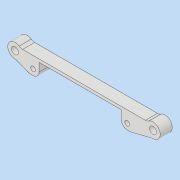
# Autodesk Inventor part: SpoolServoMount
Saved by Autodesk Inventor 2017 (Build 210142000, 142)
## iProperties
Created: 2018-04-09
Part Number: SpoolServoMount
Material: ABS Plastic
Document SubType Name: Modeling
Designer: Derek Wider
Density: 1.06 g/cm^3
Appearance: Smooth - White
Author: Derek Wider
Autodesk Inventor part; units mm, degrees
ref_plane "YZ Plane" through (0, 0, 0) normal (1, 0, 0) x (0, 1, 0)
ref_plane "XZ Plane" through (0, 0, 0) normal (0, 1, 0) x (-1, 0, 0)
ref_plane "XY Plane" through (0, 0, 0) normal (0, 0, 1) x (1, 0, 0)
sketch "Sketch1" plane through (0, 0, 0) normal (0, 0, 1) x (1, 0, 0)
  circle A0 centre (0, 0) radius 1.8415
  circle A1 centre (72.5902, 0) radius 1.8415
  line L0 (0, 0) -> (36.2951, -20.955) construction
  line L1 (0, 0) -> (41.91, 0) construction
  line L2 (36.2951, -20.955) -> (72.5902, 0) construction
  circle A2 centre (0, 0) radius 3.81
  circle A3 centre (72.5902, 0) radius 3.81
  line L3 (2.8398, 2.54) -> (69.7504, 2.54)
  line L4 (3.672, 1.016) -> (68.9182, 1.016)
  line L5 (12.7, 1.016) -> (12.7, -6.604)
  line L6 (55.88, 1.016) -> (55.88, -6.604)
  line L7 (55.88, -6.604) -> (60.96, -6.604)
  line L8 (60.96, -6.604) -> (72.22, -3.792)
  line L9 (12.7, -6.604) -> (7.62, -6.604)
  line L10 (7.62, -6.604) -> (0.3926, -3.7897)
  circle A4 centre (9.525, -3.556) radius 1.27
  circle A5 centre (59.055, -3.556) radius 1.27
  dimension "d0" = 3.683
  dimension "d1" = 41.91
  dimension "d2" = 30
  dimension "d3" = 7.62
  dimension "d4" = 5.08
  dimension "d5" = 7.62
  dimension "d6" = 2.54
  dimension "d7" = 43.18
  dimension "d8" = 4.572
  dimension "d9" = 1.524
  dimension "d10" = 1.016
  dimension "d11" = 3.175
  dimension "d12" = 3.175
  dimension "d13" = 12.7
  constraints: 22 end point, 6 centre point, 6 point on circle, 4 coincident, 4 equal length, 4 horizontal, 3 equal radius, 3 point on line, 2 horizontal alignment, 1 perpendicular, 1 vertical
  measures "d0" diameter of A0
  measures "d1" distance of L0.start L0.end
  measures "d2" angle of L0 L1
  measures "d3" diameter of A2
  measures "d4" distance of L5.end L9.end
  measures "d5" distance of L5.start L5.end
  measures "d6" diameter of A4
  measures "d7" distance between parallel lines of L6 L5
  measures "d8" distance from line of L4 A4.centre
  measures "d9" distance between parallel lines of L4 L3
  measures "d10" distance from line of point (0, 0) L4
  measures "d11" distance from line of L5 A4.centre
  measures "d12" distance from line of L6 A5.centre
  measures "d13" distance from line of L5 A2.centre
extrude "Extrusion1" add sketch "Sketch1" along normal blind 6.35
fillet "Fillet1" radius 3.175 8 edges at (2.8398, 2.54, 3.175) (12.7, -6.604, 3.175) (55.88, -6.604, 3.175) (69.7504, 2.54, 3.175) (72.22, -3.792, 3.175) (60.96, -6.604, 3.175) (7.62, -6.604, 3.175) (0.3926, -3.7897, 3.175)
body "Solid1"
